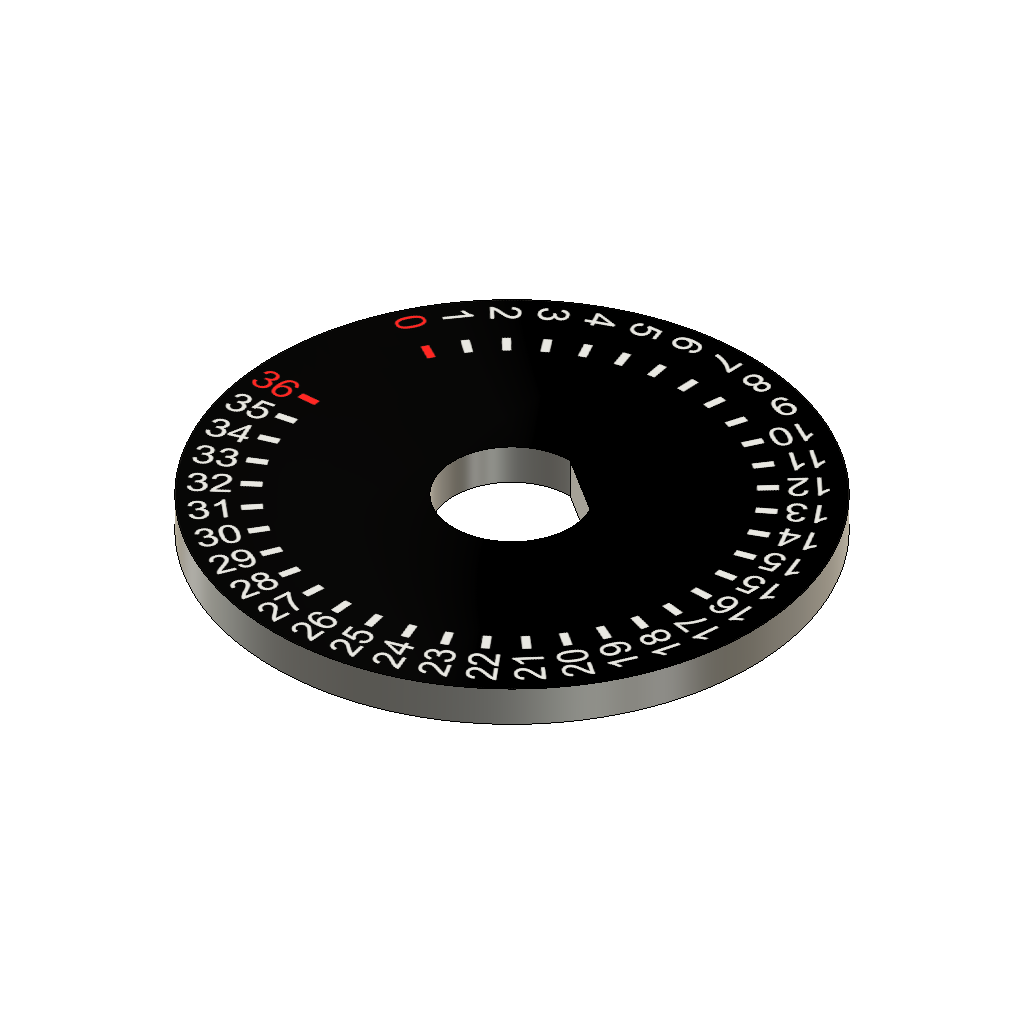
nasamoddial (Autodesk Fusion 360 design; units mm, degrees)
Autodesk Fusion 360 part; units mm, degrees
sketch "Sketch1" plane through (0, 0, 0) normal (0, 0, 1) x (1, 0, 0)
  circle A0 centre (0, 0) radius 7.8
  circle A1 centre (0, 0) radius 1.9
  line L0 (0, 1.9) -> (1.7006, 0.8474)
  point P0 (0, 1.9)
  dimension "d1" = 15.6
  dimension "d2" = 3.8
  dimension "d3" = 2
  constraint coincident A0.centre A1.centre
  constraint coincident A1 P0
  constraint coincident P0 L0.start
  constraint coincident A1 L0.end
  measures "d1" diameter of A0
  measures "d2" diameter of A1
  measures "d3" distance of P0 L0.end
extrude "Extrude1" add sketch "Sketch1" along normal blind 1 contours A0 | A1 L0 | A1 L0
sketch "Sketch2" plane through (0, 0, 1) normal (0, 0, 1) x (-1, 0, 0)
  circle A0 centre (0, 0) radius 7.8
  line L0 (0, 0) -> (-4.1053, -6.6323)
  line L1 (0, 0) -> (-6.6368, -4.0979)
  line L2 (0, 0) -> (7.8, 0)
  line L3 (0, 0) -> (7.8, 0) construction
  line L4 (0, 0) -> (6.9744, -3.4925)
  line L5 (0, 0) -> (7.8, 0) construction
  dimension "d7" = 26.55
  dimension "d10" = 26.6
  constraint coincident A0.centre L0.start
  constraint coincident A0 L0.end
  constraint coincident A0 L1.end
  constraint coincident A0 L2.end
  constraint horizontal L2
  constraint horizontal L3
  constraint horizontal L5
  measures "d7" angle of L0 L1
  measures "d10" angle of L4 L5
sketch "Sketch3" plane through (0, 0, 1) normal (0, 0, 1) x (-1, 0, 0)
  circle A0 centre (0, 0) radius 7.8
  line L0 (0, 0) -> (7.8, 0)
  line L1 (0, 0) -> (7.8, 0)
  line L2 (7.8, 0) -> (6.9743, -3.4927)
  line L3 (6.9743, -3.4927) -> (6.0802, -3.0449)
  line L4 (6.0802, -3.0449) -> (5.5437, -2.7763)
  line L5 (5.5224, -3.9677) -> (5.0352, -3.6176)
  line L6 (4.8259, -4.7907) -> (4.4001, -4.368)
  line L7 (4.008, -5.4933) -> (3.6543, -5.0086)
  line L8 (3.0893, -6.0577) -> (2.8167, -5.5232)
  line L9 (2.093, -6.4699) -> (1.9083, -5.899)
  line L10 (1.044, -6.7194) -> (0.9519, -6.1265)
  line L11 (-0.0312, -6.7999) -> (-0.0284, -6.1999)
  line L12 (-1.1056, -6.7095) -> (-1.0081, -6.1175)
  line L13 (-2.1522, -6.4504) -> (-1.9623, -5.8813)
  line L14 (-3.1447, -6.0291) -> (-2.8673, -5.4972)
  line L15 (-4.0582, -5.4563) -> (-3.7001, -4.9748)
  line L16 (-4.8696, -4.7462) -> (-4.4399, -4.3275)
  line L17 (-5.5586, -3.9169) -> (-5.0681, -3.5713)
  line L18 (-6.1078, -2.989) -> (-5.5689, -2.7253)
  line L19 (-6.5035, -1.986) -> (-5.9297, -1.8108)
  line L20 (-6.7357, -0.9331) -> (-6.1413, -0.8508)
  line L21 (-6.7985, 0.1433) -> (-6.1986, 0.1306)
  line L22 (6.3346, -4.5512) -> (5.5224, -3.9677)
  line L23 (5.5356, -5.4952) -> (4.8259, -4.7907)
  line L24 (4.5974, -6.3011) -> (4.008, -5.4933)
  line L25 (3.5436, -6.9486) -> (3.0893, -6.0577)
  line L26 (2.4008, -7.4213) -> (2.093, -6.4699)
  line L27 (1.1975, -7.7075) -> (1.044, -6.7194)
  line L28 (-0.0358, -7.7999) -> (-0.0312, -6.7999)
  line L29 (-1.2682, -7.6962) -> (-1.1056, -6.7095)
  line L30 (-2.4687, -7.399) -> (-2.1522, -6.4504)
  line L31 (-3.6072, -6.9158) -> (-3.1447, -6.0291)
  line L32 (-4.655, -6.2587) -> (-4.0582, -5.4563)
  line L33 (-5.5857, -5.4442) -> (-4.8696, -4.7462)
  line L34 (-6.376, -4.4929) -> (-5.5586, -3.9169)
  line L35 (-7.006, -3.4286) -> (-6.1078, -2.989)
  line L36 (-7.4599, -2.2781) -> (-6.5035, -1.986)
  line L37 (-7.7262, -1.0703) -> (-6.7357, -0.9331)
  line L38 (-7.7983, 0.1643) -> (-6.7985, 0.1433)
  line L39 (7.0826, -3.2674) -> (6.1746, -2.8485)
  line L40 (7.0826, -3.2674) -> (6.9743, -3.4927)
  line L41 (6.4772, -4.3459) -> (5.6468, -3.7887)
  line L42 (5.7088, -5.315) -> (4.9769, -4.6336)
  line L43 (4.797, -6.1506) -> (4.182, -5.362)
  line L44 (3.7645, -6.8314) -> (3.2819, -5.9556)
  line L45 (2.6374, -7.3406) -> (2.2992, -6.3995)
  line L46 (1.4439, -7.6652) -> (1.2588, -6.6825)
  line L47 (0.2142, -7.7971) -> (0.1867, -6.7974)
  line L48 (-1.0209, -7.7329) -> (-0.89, -6.7415)
  line L49 (-2.2304, -7.4743) -> (-1.9444, -6.5161)
  line L50 (-3.3837, -7.0278) -> (-2.9499, -6.1268)
  line L51 (-4.452, -6.4046) -> (-3.8813, -5.5835)
  line L52 (-5.4084, -5.6204) -> (-4.715, -4.8999)
  line L53 (-6.2288, -4.6949) -> (-5.4302, -4.093)
  line L54 (-6.8926, -3.6514) -> (-6.0089, -3.1832)
  line L55 (-7.3831, -2.516) -> (-6.4365, -2.1934)
  line L56 (-7.6879, -1.3174) -> (-6.7023, -1.1485)
  line L57 (-7.7995, -0.0857) -> (-6.7996, -0.0747)
  line L58 (-6.6904, 1.2161) -> (-6.1001, 1.1088)
  line L59 (-7.6743, 1.3949) -> (-6.6904, 1.2161)
  line L60 (-7.715, 1.1482) -> (-6.7259, 1.001)
  line L61 (-6.4141, 2.2583) -> (-5.8481, 2.059)
  line L62 (-7.3573, 2.5904) -> (-6.4141, 2.2583)
  line L63 (-7.4365, 2.3532) -> (-6.4831, 2.0516)
  line L64 (-5.9765, 3.2437) -> (-5.4492, 2.9575)
  line L65 (-6.8554, 3.7207) -> (-5.9765, 3.2437)
  line L66 (-6.9711, 3.4991) -> (-6.0774, 3.0505)
  line L67 (-5.3887, 4.1476) -> (-4.9132, 3.7816)
  line L68 (-6.1811, 4.7575) -> (-5.3887, 4.1476)
  line L69 (-6.3304, 4.557) -> (-5.5188, 3.9728)
  line L70 (-4.6653, 4.9472) -> (-4.2537, 4.5107)
  line L71 (-5.3514, 5.6747) -> (-4.6653, 4.9472)
  line L72 (-5.5305, 5.5003) -> (-4.8215, 4.7951)
  line L73 (-3.8247, 5.6224) -> (-3.4873, 5.1263)
  line L74 (-4.3872, 6.4492) -> (-3.8247, 5.6224)
  line L75 (-4.5916, 6.3053) -> (-4.0029, 5.4969)
  line L76 (-2.888, 6.1563) -> (-2.6331, 5.6131)
  line L77 (-3.3127, 7.0616) -> (-2.888, 6.1563)
  line L78 (-3.5373, 6.9518) -> (-3.0838, 6.0606)
  line L79 (-1.8786, 6.5354) -> (-1.7128, 5.9587)
  line L80 (-2.1548, 7.4964) -> (-1.8786, 6.5354)
  line L81 (-2.394, 7.4235) -> (-2.0871, 6.4718)
  line L82 (-0.822, 6.7501) -> (-0.7494, 6.1545)
  line L83 (-0.9428, 7.7428) -> (-0.822, 6.7501)
  line L84 (-1.1905, 7.7086) -> (-1.0379, 6.7203)
  line L85 (0.2553, 6.7952) -> (0.2328, 6.1956)
  line L86 (0.2929, 7.7945) -> (0.2553, 6.7952)
  line L87 (0.0429, 7.7999) -> (0.0374, 6.7999)
  line L88 (1.3262, 6.6694) -> (1.2091, 6.081)
  line L89 (1.5212, 7.6502) -> (1.3262, 6.6694)
  line L90 (1.2752, 7.695) -> (1.1117, 6.7085)
  line L91 (2.3637, 6.376) -> (2.1551, 5.8134)
  line L92 (2.7113, 7.3136) -> (2.3637, 6.376)
  line L93 (2.4755, 7.3967) -> (2.1581, 6.4484)
  line L94 (3.3418, 5.9222) -> (3.0469, 5.3997)
  line L95 (3.8332, 6.7931) -> (3.3418, 5.9222)
  line L96 (3.6135, 6.9125) -> (3.1503, 6.0263)
  line L97 (4.2358, 5.3196) -> (3.8621, 4.8502)
  line L98 (4.8588, 6.1018) -> (4.2358, 5.3196)
  line L99 (4.6607, 6.2544) -> (4.0632, 5.4526)
  line L100 (5.0234, 4.5832) -> (4.5802, 4.1788)
  line L101 (5.7621, 5.2572) -> (5.0234, 4.5832)
  line L102 (5.5907, 5.4391) -> (4.874, 4.7418)
  line L103 (5.6847, 3.7315) -> (5.1831, 3.4023)
  line L104 (6.5207, 4.2803) -> (5.6847, 3.7315)
  line L105 (6.3801, 4.4871) -> (5.5622, 3.9118)
  line L106 (6.203, 2.7861) -> (5.6557, 2.5403)
  line L107 (7.1153, 3.1958) -> (6.203, 2.7861)
  line L108 (7.0092, 3.4222) -> (6.1106, 2.9834)
  line L109 (6.5654, 1.7706) -> (5.9861, 1.6144)
  line L110 (7.5309, 2.031) -> (6.5654, 1.7706)
  line L111 (7.462, 2.2713) -> (6.5053, 1.9801)
  line L112 (6.7628, 0.7106) -> (6.1661, 0.6479)
  line L113 (7.7573, 0.8151) -> (6.7628, 0.7106)
  line L114 (7.7272, 1.0633) -> (6.7365, 0.927)
  dimension "d12" = 3.589
  dimension "d14" = 1
  dimension "d15" = 0.6
  dimension "d17" = -327.4
  dimension "d28" = 1
  dimension "d29" = 0.25
  dimension "d30" = 0.5
  dimension "d31" = 0
  dimension "d32" = 0.5
  dimension "d33" = 0
  dimension "d34" = 0.5
  dimension "d35" = 0
  dimension "d36" = 0.5
  dimension "d37" = 0
  dimension "d38" = 0.5
  dimension "d39" = 0
  dimension "d40" = 0.5
  dimension "d41" = 0
  dimension "d42" = 0.5
  dimension "d43" = 0
  dimension "d44" = 0.5
  dimension "d45" = 0
  dimension "d46" = 0.5
  dimension "d47" = 0
  dimension "d48" = 0.5
  dimension "d49" = 0
  dimension "d50" = 0.5
  dimension "d51" = 0
  dimension "d52" = 0.5
  dimension "d53" = 0
  dimension "d54" = 0.5
  dimension "d55" = 0
  constraint coincident A0.centre L0.start
  constraint coincident A0 L0.end
  constraint horizontal L0
  constraint coincident A0 L2.end
  constraint perpendicular A0 L3
  constraint parallel L3 L4
  constraint coincident A0 L39.start
  constraint perpendicular A0 L39
  measures "d12" distance of L0.end L2.end
  measures "d14" distance of L2.end L3.end
  measures "d15" distance of L3.end L4.end
  measures "d28" distance of L39.start L39.end
  measures "d29" distance of L2.end L39.start
sketch "Sketch4" plane through (0, 0, 1) normal (0, 0, 1) x (-1, 0, 0)
  circle A0 centre (0, 0) radius 7.8
extrude "Extrude2" cut sketch "Sketch1" along normal blind 1.5 contours A1 L0 picked at (0.031, -0.6295)
emboss "Emboss1" [rolled back] depth -0.01 horizontal distance 0 vertical distance 0 rotation angle 0
equation "d31 = '0 -'"
equation "d33 = '1 -'"
equation "d35 = '2'"
equation "d37 = '3'"
equation "d39 = '4'"
equation "d41 = '5'"
equation "d43 = '6'"
equation "d45 = '8'"
equation "d47 = '9'"
equation "d49 = '10'"
equation "d51 = '11'"
equation "d53 = '12'"
equation "d55 = '13'"
